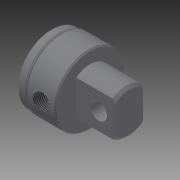
# Autodesk Inventor part: 17P0000_rear_head
Saved by Autodesk Inventor 2014 (Build 180170000, 170)
## iProperties
Created: 2014-01-18
Part Number: 17P0000_rear_head
Material: Generic
Catalog Web Link: www.cadenas.de
Description: Rear Head-Original Line - Standard Air Cylinders
Vendor: BIMBA
Document SubType Name: Standard Catalog Part
Designer: Andrew Toennies
Manufacturer: BIMBA
Density: 1 g/cm^3
Appearance: RGB(211.00000262260440,211.00000262260440,211.00000262260440)
Category: PARTsolutions
Company: BIMBA
Title: 17P0000_rear_head
Author: Cadenas PARTsolutions
Comments: Original Line - Standard Air Cylinders
PSOL_IDENT_0: {$CADENAS_DATA\23d-libs\bimba\bimba\bimba_imperial\bimba_full_line\original_line_cylinders\standard_
PSOL_IDENT_1: air_cylinders\rear_head.prj},229 {VTYP=3D},{NB=17P0000_rear_head},{LINA=17P0000_rear_head},{NN=Rear
PSOL_IDENT_2: Head},{DATE=05.09.2013 09:05:50},{GEOMDATE=05.09.2013 11:04:00},{VERSION=},{LINEID=80},{LINESUBID=-1
PSOL_IDENT_3: },{WBVAR=MNT,ACTING,DER,Q,T1,T2,T3,T4,TRIM,Y,K,MB,CUSH,FBON}  {NB=17P0000_rear_head},{LINA=17P0000_r
PSOL_IDENT_4: ear_head},{KT=DUMMY},{PN=17P0000},{BORE=1.50000},{BOREPN=17},{MNT=P},{MNTALG='' , 'Front Nose' , 'P'
PSOL_IDENT_5: , 'Rear Pivot' , 'S' , 'Built-in Valve S' , 'DX' , 'Double End' , 'A' , 'Adjustable Stroke' , 'M' ,
PSOL_IDENT_6: 'Manual Valve' , 'BR' , 'Rear Block' , 'BRT' , 'Rear Trunnion'},{ACTING=},{ACTINGALG= '' , 'Single
PSOL_IDENT_7: Acting' },{DER=},{DERALG= '' , 'Standard' },{Q=},{T1=},{T2=},{T3=},{T4=},{TRIM=0},{Y=},{K=},{KALG= ''
PSOL_IDENT_8: , 'without K', 'K', 'with K' },{MB=0},{A1=1.7500},{A1N=0.6880},{A1P=1.7500},{A1B=1.3750},{A1S=1.5000
PSOL_IDENT_9: },{A2=0.25},{A2N=0.2500},{A3=0.0400},{D1=1.5565},{D1N=1.5565},{D1P=1.5565},{D1B=1.5800},{D2=1.5115},
PSOL_IDENT_10: {C1=0.0300},{C2=0.0300},{NDM=0.4050},{TAB=NPT},{NDMDP=0.2730},{D3=0.3440},{A4=0.2500},{A5=0.8700},{D
PSOL_IDENT_11: 4=0.9730},{A6=0.2500},{A7=0.6250},{A8=0.0000},{D5=0.0000},{D6=0.5320},{A9=0.7320},{NDM2=0.0000},{TAB
PSOL_IDENT_12: 2=-},{C11=0.0300},{C22=0.0000},{C33=0.0000},{C44=0.0300},{A10=0.6170},{A11=0.0000},{NDM3=0.4050},{ND
PSOL_IDENT_13: M3N=0.4050},{NDM3B=0.5400},{TAB3=NPT},{TAB3N=NPT},{TAB3B=NPT},{A12=0.562},{A12N=0.5620},{A12B=0.7500
PSOL_IDENT_14: },{A13=1.3750},{D7=0.3775},{D8=1.0000},{A14=0.0000},{A15=0.0000},{D9=0.0000},{R1=0.0000},{X1=0.9690}
PSOL_IDENT_15: ,{X2=0.2500},{CX=0.0600},{CC=0.0000},{CON=1},{S1=1.7500},{DB=0.4380},{X1B=0.9730},{X2B=0.2500},{A8B=
PSOL_IDENT_16: 0.1250},{A9B=1.0620},{MODEL=1},{NDM4=0.2500},{TAB4=UNC},{NDM4DP=0.5000},{BC=1.7500},{B1=0.8750},{B2=
PSOL_IDENT_17: 0.3800},{B3=0.5000},{ON=0},{ON2=1},{G1=0.0000},{G2=0.0000},{G3=0.0000},{G4=0.0000},{GD=0.0000},{G5=0
PSOL_IDENT_18: .0000},{G6=0.0000},{RON=0},{H1=1.6160},{H2=1.5800},{H3=0.1250},{H4=0.1250},{H5=1.5300},{H6=0.8120},{
PSOL_IDENT_19: F=0.6240},{PNUT=0.0000},{CUSH=0},{CC11=0.397},{CC111=0.3965},{CC22=0.5625},{CC33=0.3050},{CC44=0.625
PSOL_IDENT_20: 0},{CC55=0.8750},{CD1=0.2650},{CD2=0.1980},{CD3=0.1345},{CNDM3=0.2500},{CTAB3=UNS},{OLEN=1.3750},{OD=
PSOL_IDENT_21: 0.5025},{STDIS=0.3184},{STDIS1=0.3184},{BUSHCON=D-624},{BUSHL=0.7500},{FBON=0},{LCD=0.0000}
CNS_NN: Rear Head
CNS_NT: Original Line - Standard Air Cylinders
CNS_NB: 17P0000_rear_head
CNS_NBSYN: $PN._rear_head
CNS_LINA: 17P0000_rear_head
CNS_PN: 17P0000
CNS_BORE: 1.50000
CNS_BOREPN: 17
CNS_MNT: Rear Pivot
CNS_MNTALG: '' , 'Front Nose' , 'P' , 'Rear Pivot' , 'S' , 'Built-in Valve S' , 'DX' , 'Double End' , 'A' , 'Adjustable Stroke' , 'M' , 'Manual Valve' , 'BR' , 'Rear Block' , 'BRT' , 'Rear Trunnion'
CNS_ACTING: Single Acting
CNS_ACTINGALG: '' , 'Single Acting'
CNS_DER: Standard
CNS_DERALG: '' , 'Standard'
CNS_Q: Without Side Ported Rear Head
CNS_T1: without T1
CNS_T2: without T2
CNS_T3: without T3
CNS_T4: without T4
CNS_TRIM: 0
CNS_Y: without Pivot Bushing
CNS_K: without K
CNS_KALG: '', 'without K', 'K', 'with K'
CNS_MB: 0
CNS_A1: 1.7500
CNS_A1N: 0.6880
CNS_A1P: 1.7500
CNS_A1B: 1.3750
CNS_A1S: 1.5000
CNS_A2: 0.250
CNS_A2N: 0.2500
CNS_A3: 0.0400
CNS_D1: 1.5565
CNS_D1N: 1.5565
CNS_D1P: 1.5565
CNS_D1B: 1.5800
CNS_D2: 1.5115
CNS_C1: 0.0300
CNS_C2: 0.0300
CNS_NDM: 0.4050
CNS_TAB: NPT
CNS_NDMDP: 0.2730
CNS_D3: 0.3440
CNS_A4: 0.2500
CNS_A5: 0.8700
CNS_D4: 0.9730
CNS_A6: 0.2500
CNS_A7: 0.6250
CNS_A8: 0.0000
CNS_D5: 0.0000
CNS_D6: 0.5320
CNS_A9: 0.7320
CNS_NDM2: 0.0000
CNS_TAB2: -
CNS_C11: 0.0300
CNS_C22: 0.0000
CNS_C33: 0.0000
CNS_C44: 0.0300
CNS_A10: 0.6170
CNS_A11: 0.0000
CNS_NDM3: 0.4050
CNS_NDM3N: 0.4050
CNS_NDM3B: 0.5400
CNS_TAB3: NPT
CNS_TAB3N: NPT
CNS_TAB3B: NPT
CNS_A12: 0.562
CNS_A12N: 0.5620
CNS_A12B: 0.7500
CNS_A13: 1.3750
CNS_D7: 0.3775
CNS_D8: 1.0000
CNS_A14: 0.0000
CNS_A15: 0.0000
CNS_D9: 0.0000
CNS_R1: 0.0000
CNS_X1: 0.9690
CNS_X2: 0.2500
CNS_CX: 0.0600
CNS_CC: 0.0000
CNS_CON: 1
CNS_S1: 1.7500
CNS_DB: 0.4380
CNS_X1B: 0.9730
CNS_X2B: 0.2500
CNS_A8B: 0.1250
CNS_A9B: 1.0620
CNS_MODEL: 1
CNS_NDM4: 0.2500
CNS_TAB4: UNC
CNS_NDM4DP: 0.5000
CNS_BC: 1.7500
CNS_B1: 0.8750
CNS_B2: 0.3800
CNS_B3: 0.5000
CNS_ON: 0
CNS_ON2: 1
CNS_G1: 0.0000
CNS_G2: 0.0000
CNS_G3: 0.0000
CNS_G4: 0.0000
CNS_GD: 0.0000
CNS_G5: 0.0000
CNS_G6: 0.0000
CNS_RON: 0
CNS_H1: 1.6160
CNS_H2: 1.5800
CNS_H3: 0.1250
CNS_H4: 0.1250
CNS_H5: 1.5300
CNS_H6: 0.8120
CNS_F: 0.6240
CNS_PNUT: 0.0000
CNS_CUSH: 0
CNS_CC11: 0.397
CNS_CC111: 0.3965
CNS_CC22: 0.5625
CNS_CC33: 0.3050
CNS_CC44: 0.6250
CNS_CC55: 0.8750
CNS_CD1: 0.2650
CNS_CD2: 0.1980
CNS_CD3: 0.1345
CNS_CNDM3: 0.2500
CNS_CTAB3: UNS
CNS_OLEN: 1.3750
CNS_OD: 0.5025
CNS_STDIS: 0.3184
CNS_STDIS1: 0.3184
CNS_BUSHCON: D-624
CNS_BUSHL: 0.7500
CNS_FBON: 0
CNS_LCD: 0.0000
SUPPLIER: BIMBA
ARTICLENO: 17P0000_rear_head
BOMINFO: 17P0000_rear_head
CREATOR: CADENAS GmbH
Autodesk Inventor part; units mm, degrees
ref_plane "YZ Plane" through (0, 0, 0) normal (1, 0, 0) x (0, 1, 0)
ref_plane "XZ Plane" through (0, 0, 0) normal (0, 1, 0) x (-1, 0, 0)
ref_plane "XY Plane" through (0, 0, 0) normal (0, 0, 1) x (1, 0, 0)
sketch "Sketch_18" plane through (0, 0, 0) normal (0, 0, 1) x (1, 0, 0)
  line L0 (22.225, 0) -> (0, 0)
  line L1 (0, 0) -> (0, 18.434)
  line L2 (0, 18.434) -> (0.762, 19.196)
  line L3 (0.762, 19.196) -> (4.318, 19.196)
  line L4 (4.318, 19.196) -> (5.334, 18.1801)
  line L5 (5.334, 18.1801) -> (6.35, 18.1801)
  line L6 (6.35, 18.1801) -> (6.35, 19.7675)
  line L7 (6.35, 19.7675) -> (21.463, 19.7675)
  line L8 (21.463, 19.7675) -> (22.225, 19.0055)
  line L9 (22.225, 19.0055) -> (22.225, 0)
  line L10 (22.225, 0) -> (0, 0)
  constraints: 22 end point
revolve "Revolution1" add sketch "Sketch_18" angle 360 about axis through (22.225, 0, 0) along (1, 0, 0)
sketch "Sketch_21" plane through (0, 0, 0) normal (0, 0, 1) x (1, 0, 0)
  line L0 (44.45, 0) -> (22.225, 0)
  line L1 (22.225, 0) -> (22.225, 12.7)
  line L2 (22.225, 12.7) -> (42.926, 12.7)
  line L3 (42.926, 12.7) -> (44.45, 11.176)
  line L4 (44.45, 11.176) -> (44.45, 0)
  line L5 (44.45, 0) -> (22.225, 0)
  constraints: 12 end point
revolve "Revolution2" add sketch "Sketch_21" angle 360 about axis through (44.45, 0, 0) along (1, 0, 0)
sketch "Sketch_9" plane through (44.45, 0, 0) normal (1, 0, 0) x (0, 0, -1)
  line L0 (-39.5351, -79.0702) -> (39.5351, -79.0702)
  line L1 (39.5351, -79.0702) -> (39.5351, 79.0702)
  line L2 (39.5351, 79.0702) -> (-39.5351, 79.0702)
  line L3 (-39.5351, 79.0702) -> (-39.5351, -79.0702)
  line L4 (-7.8359, -39.5351) -> (7.8359, -39.5351)
  line L5 (7.8359, -39.5351) -> (7.8359, 39.5351)
  line L6 (7.8359, 39.5351) -> (-7.8359, 39.5351)
  line L7 (-7.8359, 39.5351) -> (-7.8359, -39.5351)
  constraints: 16 end point
extrude "Extrusion1" cut sketch "Sketch_9" against normal blind 22.225
sketch "Sketch4" plane through (0, 0, 0) normal (-1, 0, 0) x (0, 0, 1)
  point P0 (0, 0)
hole "Hole1" at (0, 0, 0) direction (1, 0, 0) diameter 13.5128 depth 20.4521 tip angle 120
sketch "Sketch_68" plane through (0, 0, 0) normal (0, 0.9998477, 0.0174524) x (1, 0, 0)
  line L0 (14.2748, -19.7675) -> (14.2748, 0)
  line L1 (14.2748, 0) -> (18.8978, 0)
  line L2 (18.8978, 0) -> (18.8978, -12.8333)
  line L3 (18.8978, -12.8333) -> (19.1143, -19.7675)
  line L4 (19.1143, -19.7675) -> (14.2748, -19.7675)
  line L5 (14.2748, -19.7675) -> (14.2748, 0)
  constraints: 12 end point
revolve "Revolution3" cut sketch "Sketch_68" angle 360 about axis through (14.2748, -0.345, 19.7645) along (0, -0.0174524, 0.9998477)
thread "Thread1" size "1/8" designation "1/8 - 27 NPT" standard "NPT" full length
sketch "Sketch_20" plane through (0, 0, 0) normal (0, 0, 1) x (1, 0, 0)
  line L0 (6.35, 0) -> (0, 0)
  line L1 (0, 0) -> (0, 12.3063)
  line L2 (0, 12.3063) -> (6.35, 12.3063)
  line L3 (6.35, 12.3063) -> (6.35, 0)
  line L4 (6.35, 0) -> (0, 0)
  constraints: 10 end point
revolve "Revolution4" cut sketch "Sketch_20" angle 360 about axis through (6.35, 0, 0) along (1, 0, 0)
sketch "Sketch_24" plane through (0, 0, 0) normal (0, 0, 1) x (1, 0, 0)
  line L0 (6.35, 0) -> (5.334, 0)
  line L1 (5.2675, 19.6834) -> (6.2166, 18.7343)
  arc A0 (6.2166, 18.5547) -> (6.2166, 18.7343) centre (6.1268, 18.6445) ccw
  line L2 (6.2166, 18.5547) -> (5.842, 18.1801)
  line L3 (5.842, 18.1801) -> (5.334, 18.1801)
  line L4 (5.334, 18.1801) -> (5.334, 17.9261)
  line L5 (5.334, 17.9261) -> (6.35, 17.9261)
  line L6 (6.35, 17.9261) -> (6.35, 18.8883)
  line L7 (6.35, 18.8883) -> (5.4707, 19.7675)
  line L8 (5.4707, 19.7675) -> (5.2675, 19.7675)
  line L9 (5.2675, 19.7675) -> (5.2675, 19.6834)
  constraints: 20 end point, 2 point on circle, 1 centre point
revolve "Revolution5" add sketch "Sketch_24" angle 360 about axis through (6.35, 0, 0) along (1, 0, 0)
sketch "Sketch_43" plane through (0, 0, 0) normal (0, 0, 1) x (1, 0, 0)
  circle A0 centre (34.925, 0) radius 4.7942
  constraints: 1 centre point
extrude "Extrusion2" cut sketch "Sketch_43" along normal mid plane 23.5077
ref_plane "f_XY" through (22.225, 0, 0) normal (0, 0, 1) x (1, 0, 0)
ref_plane "f_YZ" through (22.225, 0, 0) normal (1, 0, 0) x (0, 1, 0)
ref_plane "f_ZX" through (22.225, 0, 0) normal (0, 1, 0) x (0, 0, 1)
ref_plane "lovra1_XY" through (38.1, 0, 0) normal (1, 0, 0) x (0, 0, -1)
ref_plane "lovra1_YZ" through (38.1, 0, 0) normal (0, 0, -1) x (0, 1, 0)
ref_plane "lovra1_ZX" through (38.1, 0, 0) normal (0, 1, 0) x (1, 0, 0)
ref_plane "lovra2_XY" through (38.1, 11.049, 0) normal (1, 0, 0) x (0, 0, -1)
ref_plane "lovra2_YZ" through (38.1, 11.049, 0) normal (0, 0, -1) x (0, 1, 0)
ref_plane "lovra2_ZX" through (38.1, 11.049, 0) normal (0, 1, 0) x (1, 0, 0)
ref_plane "lovra21_XY" through (0, 0, 5.2705) normal (1, 0, 0) x (0, 0, -1)
ref_plane "lovra21_YZ" through (0, 0, 5.2705) normal (0, 0, -1) x (0, 1, 0)
ref_plane "lovra21_ZX" through (0, 0, 5.2705) normal (0, 1, 0) x (1, 0, 0)
ref_plane "lovra22_XY" through (0, 0, -5.2705) normal (1, 0, 0) x (0, 0, -1)
ref_plane "lovra22_YZ" through (0, 0, -5.2705) normal (0, 0, -1) x (0, 1, 0)
ref_plane "lovra22_ZX" through (0, 0, -5.2705) normal (0, 1, 0) x (1, 0, 0)
ref_plane "lovra3_XY" through (38.1, -11.049, 0) normal (1, 0, 0) x (0, 0, -1)
ref_plane "lovra3_YZ" through (38.1, -11.049, 0) normal (0, 0, -1) x (0, 1, 0)
ref_plane "lovra3_ZX" through (38.1, -11.049, 0) normal (0, 1, 0) x (1, 0, 0)
ref_plane "olen_XY" through (34.925, 0, 0) normal (1, 0, 0) x (0, 0, -1)
ref_plane "olen_YZ" through (34.925, 0, 0) normal (0, 0, -1) x (0, 1, 0)
ref_plane "olen_ZX" through (34.925, 0, 0) normal (0, 1, 0) x (1, 0, 0)
ref_plane "p1_XY" through (44.45, 0, 7.8359) normal (1, 0, 0) x (0, 0, -1)
ref_plane "p1_YZ" through (44.45, 0, 7.8359) normal (0, 0, -1) x (0, 1, 0)
ref_plane "p1_ZX" through (44.45, 0, 7.8359) normal (0, 1, 0) x (1, 0, 0)
ref_plane "p2_XY" through (44.45, 0, -7.8359) normal (1, 0, 0) x (0, 0, -1)
ref_plane "p2_YZ" through (44.45, 0, -7.8359) normal (0, 0, -1) x (0, 1, 0)
ref_plane "p2_ZX" through (44.45, 0, -7.8359) normal (0, 1, 0) x (1, 0, 0)
ref_plane "port_XY" through (14.2748, 0, 0) normal (0, 0, 1) x (1, 0, 0)
ref_plane "port_YZ" through (14.2748, 0, 0) normal (1, 0, 0) x (0, 1, 0)
ref_plane "port_ZX" through (14.2748, 0, 0) normal (0, 1, 0) x (0, 0, 1)
ref_plane "port2_XY" through (44.45, 0, 0) normal (1, 0, 0) x (0, 0, -1)
ref_plane "port2_YZ" through (44.45, 0, 0) normal (0, 0, -1) x (0, 1, 0)
ref_plane "port2_ZX" through (44.45, 0, 0) normal (0, 1, 0) x (1, 0, 0)
ref_plane "thd1_XY" through (44.45, 0, 0) normal (1, 0, 0) x (0, 0, -1)
ref_plane "thd1_YZ" through (44.45, 0, 0) normal (0, 0, -1) x (0, 1, 0)
ref_plane "thd1_ZX" through (44.45, 0, 0) normal (0, 1, 0) x (1, 0, 0)
ref_plane "thd2_XY" through (44.45, 0, 0) normal (1, 0, 0) x (0, 0, -1)
ref_plane "thd2_YZ" through (44.45, 0, 0) normal (0, 0, -1) x (0, 1, 0)
ref_plane "thd2_ZX" through (44.45, 0, 0) normal (0, 1, 0) x (1, 0, 0)
ref_plane "to_mounting_bracket_XY" through (22.225, 0, 0) normal (1, 0, 0) x (0, 0, -1)
ref_plane "to_mounting_bracket_YZ" through (22.225, 0, 0) normal (0, 0, -1) x (0, 1, 0)
ref_plane "to_mounting_bracket_ZX" through (22.225, 0, 0) normal (0, 1, 0) x (1, 0, 0)
ref_plane "to_nut_XY" through (0, 0, 0) normal (1, 0, 0) x (0, 0, -1)
ref_plane "to_nut_YZ" through (0, 0, 0) normal (0, 0, -1) x (0, 1, 0)
ref_plane "to_nut_ZX" through (0, 0, 0) normal (0, 1, 0) x (1, 0, 0)
ref_plane "to_pin_XY" through (34.925, 0, 0) normal (0, 0, 1) x (1, 0, 0)
ref_plane "to_pin_YZ" through (34.925, 0, 0) normal (1, 0, 0) x (0, 1, 0)
ref_plane "to_pin_ZX" through (34.925, 0, 0) normal (0, 1, 0) x (0, 0, 1)
ref_plane "to_screw_XY" through (14.2748, 14.2875, -10.0838) normal (0, 1, 0) x (1, 0, 0)
ref_plane "to_screw_YZ" through (14.2748, 14.2875, -10.0838) normal (1, 0, 0) x (0, 0, -1)
ref_plane "to_screw_ZX" through (14.2748, 14.2875, -10.0838) normal (0, 0, -1) x (0, 1, 0)
ref_plane "to_tube_XY" through (5.334, 0, 0) normal (1, 0, 0) x (0, 0, -1)
ref_plane "to_tube_YZ" through (5.334, 0, 0) normal (0, 0, -1) x (0, 1, 0)
ref_plane "to_tube_ZX" through (5.334, 0, 0) normal (0, 1, 0) x (1, 0, 0)
body "Solid1"
